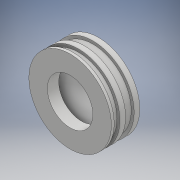
# Autodesk Inventor part: Valvula
Saved by Autodesk Inventor 2018.3 (Build 223284000, 284)
## iProperties
Created: 2019-02-26
Part Number: Valvula
Material: Generic
Document SubType Name: Modeling
Designer: Mario
Density: 1 g/cm^3
Appearance: Default
Author: Mario
Autodesk Inventor part; units mm, degrees
ref_plane "YZ Plane" through (0, 0, 0) normal (1, 0, 0) x (0, 1, 0)
ref_plane "XZ Plane" through (0, 0, 0) normal (0, 1, 0) x (-1, 0, 0)
ref_plane "XY Plane" through (0, 0, 0) normal (0, 0, 1) x (1, 0, 0)
sketch "Sketch1" plane through (0, 0, 0) normal (0, 1, 0) x (-1, 0, 0)
  circle A0 centre (0, 0) radius 14.5
  dimension "d0" = 29
  constraints: 1 centre point, 1 coincident
  measures "d0" diameter of A0
extrude "Extrusion1" add sketch "Sketch1" along normal blind 14
sketch "Sketch2" plane through (0, 0, 0) normal (1, 0, 0) x (0, 1, 0)
  line L0 (14, -14.5) -> (14, 14.5) projected
  line L1 (14, 0) -> (14, -25)
  line L2 (14, -25) -> (7.1034, -25)
  line L3 (7.1034, -25) -> (14, 0)
  line L4 (5, -14.5) -> (5, -13.5)
  line L5 (5, -13.5) -> (8, -13.5)
  line L6 (8, -13.5) -> (8, -14.5)
  line L7 (8, -14.5) -> (5, -14.5)
  line L8 (1, -13.5) -> (3, -13.5)
  line L9 (3, -13.5) -> (3, -14.5)
  line L10 (3, -14.5) -> (1, -14.5)
  line L11 (1, -14.5) -> (1, -13.5)
  line L12 (0, 14.5) -> (0, -14.5) projected
  line L13 (0, -14.5) -> (14, -14.5) projected
  line L14 (-2.8, 0) -> (16.8, 0) projected
  point P0 (0, 0)
  point P1 (10, -14.5)
  dimension "d3" = 1
  dimension "d4" = 3
  dimension "d5" = 2
  dimension "d6" = 1
  dimension "d7" = 2
  dimension "d8" = 1
  dimension "d9" = 2
  dimension "d10" = 25
  constraints: 22 end point, 5 perpendicular, 2 collinear, 2 parallel, 2 point on line, 2 vertical, 1 horizontal, 1 midpoint
  measures "d3" distance of L5.end L6.end
  measures "d4" distance of L4.end L5.end
  measures "d5" distance of L9.end L10.end
  measures "d6" distance of L8.end L9.end
  measures "d7" distance between parallel lines of L4 L9
  measures "d8" distance from line of L10.end L12
  measures "d9" distance of L6.end point (10, -14.5)
  measures "d10" distance from line of L1.start L2
revolve "Revolution1" cut sketch "Sketch2" angle 360 about axis through (0, -10, 0) along (0, 1, 0) contours L13 L3 L0 | L1 L2 L3 L13 | L7 L4 L5 L6 | L11 L8 L9 L10
sketch "Sketch3" plane through (0, 0, 0) normal (1, 0, 0) x (0, 1, 0)
  line L0 (0, 0) -> (0, 8)
  line L1 (0, 8) -> (4, 8)
  line L2 (4, 8) -> (4, 13.7374)
  line L3 (4, 13.7374) -> (9, 0)
  line L4 (9, 0) -> (0, 0)
  line L5 (9, 0) -> (9, 10.144) construction
  line L6 (0, 14.5) -> (0, -14.5) construction
  line L7 (-2.8, 0) -> (16.8, 0) construction
  point P0 (0, 0)
  dimension "d12" = 8
  dimension "d13" = 4
  dimension "d14" = 5
  dimension "d15" = 20
  dimension "d19" = 10.144
  constraints: 12 end point, 3 vertical, 2 collinear, 1 horizontal, 1 parallel
  measures "d12" distance between parallel lines of L4 L1
  measures "d13" distance of L0.end L1.end
  measures "d14" distance from line of L3.end L2
  measures "d15" angle of L5 L3
  measures "d19" distance from line of L5.end L7
revolve "Revolution2" cut sketch "Sketch3" angle 360 about axis through (0, -10, 0) along (0, 1, 0)
body "Solid1"
